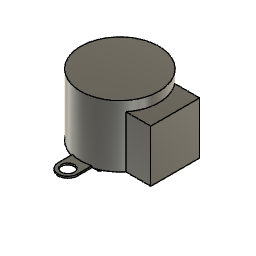
Moteur_Boule v1 (Autodesk Fusion 360 design; units mm, degrees)
Autodesk Fusion 360 part; units mm, degrees
sketch "Esquisse1" plane through (0, 0, 0) normal (0, 0, 1) x (1, 0, 0)
  circle A0 centre (0, 0) radius 12
  line L0 (9, 0) -> (17, 0)
  line L1 (17, -7.5) -> (9, -7.5)
  line L2 (9, -7.5) -> (9, 7.5)
  line L3 (9, 7.5) -> (17, 7.5)
  line L4 (17, 7.5) -> (17, -7.5)
  dimension "d1" = 24
  dimension "d3" = 8
  dimension "d4" = 17
  dimension "d5" = 15
  dimension "d8" = 7.5
  dimension "d9" = 8
  constraint coincident A0.centre origin
  constraint horizontal L0
  constraint horizontal L1
  constraint vertical L2
  constraint horizontal L3
  constraint vertical L4
  constraint collinear A0.centre L0.start L0.end
  constraint collinear L0.end L1.start L3.end
  measures "d1" diameter of A0
  measures "d3" distance of L0.start L0.end
  measures "d4" distance of A0.centre L0.end
  measures "d5" distance of L1 L3
  measures "d8" distance of L0 L1
  measures "d9" distance of L2.end L3.end
extrude "Extrusion1" add sketch "Esquisse1" along normal blind 16
sketch "Esquisse2" plane through (0, 0, 16) normal (0, 0, 1) x (-1, 0, 0)
  arc A0 (-9.3675, -7.5) -> (-9.3675, 7.5) centre (0, 0) ccw
  line L0 (-9.3675, 7.5) -> (-17, 7.5)
  line L1 (-17, 7.5) -> (-17, -7.5)
  line L2 (-17, -7.5) -> (-9.3675, -7.5)
  circle A1 centre (0, 0) radius 12
  constraint concentric A0 A1
extrude "Extrusion2" add sketch "Esquisse2" along normal blind 3 contours A0 A1
sketch "Esquisse5" plane through (0, 0, 0) normal (0, 0, -1) x (1, 0, 0)
  arc A0 (9.3675, 7.5) -> (9.3675, -7.5) centre (0, 0) ccw
  line L0 (9.3675, -7.5) -> (17, -7.5)
  line L1 (17, -7.5) -> (17, 7.5)
  line L2 (17, 7.5) -> (9.3675, 7.5)
  circle A1 centre (0, 16) radius 2
  line L3 (0, 0) -> (12, 0)
  circle A2 centre (0, 0) radius 12
  line L4 (3, 16) -> (3, 11.619)
  line L5 (0, 0) -> (0, 19)
  arc A3 (-3, -16) -> (0, -19) centre (0, -16) ccw
  line L6 (3, -16) -> (3, -11.619)
  circle A4 centre (0, -16) radius 2
  line L7 (-3, 16) -> (-3, 11.619)
  arc A5 (0, -19) -> (3, -16) centre (0, -16) ccw
  arc A6 (0, 19) -> (-3, 16) centre (0, 16) ccw
  line L8 (-3, 16) -> (3, 16)
  arc A7 (3, 16) -> (0, 19) centre (0, 16) ccw
  line L9 (-3, -16) -> (-3, -11.619)
  point P0 (0, 12)
  dimension "d27" = 19
  dimension "d28" = 4
  dimension "d29" = 24
  dimension "d30" = 3
  constraint coincident A0.centre L3.start
  constraint vertical L5
  constraint coincident A1.centre L5
  constraint coincident P0 L5
  constraint perpendicular L3 L5
  constraint coincident A1.centre A6.centre
  constraint perpendicular L5 L8
  constraint coincident L4.end A2
  constraint tangent L4 A7
  constraint coincident L7.end A2
  constraint tangent L7 A6
  constraint perpendicular L7 L8
  constraint symmetric A3.end L5.end L3
  constraint symmetric A1 L3 A4
  constraint symmetric L6.start L4.start L3
  constraint symmetric L3 A5 A7
  constraint symmetric A3.start L7.start L3
  constraint symmetric L3 A3 A6
  constraint symmetric L4.end L6.end L3
  constraint symmetric L7.end L9.end L3
  measures "d27" distance of A0.centre L5.end
  measures "d28" diameter of A1
  measures "d29" diameter of A2
  measures "d30" distance of L8 A7
extrude "Extrusion4" add sketch "Esquisse5" against normal blind 0.5 contours A0 A1 A2 L4 L5 L8 | A0 A1 A2 L5 L7 L8 | A1 L5 L8 A7 | A1 L5 A6 L8 | A0 A2 A3 L6 A5 L9
sketch "Esquisse6" plane through (0, 0, 0) normal (0, 0, -1) x (1, 0, 0)
  circle A0 centre (0, -16) radius 2
  circle A1 centre (0, 16) radius 2
  arc A2 (3, -11.619) -> (9.3675, -7.5) centre (0, 0) ccw
  line L0 (9.3675, -7.5) -> (17, -7.5)
  line L1 (17, -7.5) -> (17, 7.5)
  line L2 (17, 7.5) -> (9.3675, 7.5)
  arc A3 (9.3675, 7.5) -> (3, 11.619) centre (0, 0) ccw
  line L3 (3, 11.619) -> (3, 16)
  arc A4 (3, 16) -> (-3, 16) centre (0, 16) ccw
  line L4 (-3, 16) -> (-3, 11.619)
  arc A5 (-3, 11.619) -> (-3, -11.619) centre (0, 0) ccw
  line L5 (-3, -11.619) -> (-3, -16)
  arc A6 (-3, -16) -> (3, -16) centre (0, -16) ccw
  line L6 (3, -16) -> (3, -11.619)
  circle A7 centre (-7, 0) radius 4
  line L7 (-7, 0) -> (-12, 0)
  dimension "d33" = 8
  dimension "d34" = 5
  constraint coincident A7.centre L7.start
  constraint midpoint A5 L7.end
  constraint horizontal L7
  measures "d33" diameter of A7
  measures "d34" distance of A7.centre L7.end
extrude "Extrusion5" add sketch "Esquisse6" along normal blind 1 contours A7
sketch "Esquisse7" plane through (0, 0, -1) normal (0, 0, -1) x (1, 0, 0)
  circle A0 centre (-7, 0) radius 4
  circle A1 centre (-7, 0) radius 2.5
  dimension "d37" = 5
  constraint concentric A0 A1
  measures "d37" diameter of A1
extrude "Extrusion6" add sketch "Esquisse7" along normal blind 9 contours A1
sketch "Esquisse8" plane through (0, 0, -10) normal (0, 0, -1) x (1, 0, 0)
  circle A0 centre (-7, 0) radius 2.5
  line L0 (-7, 0) -> (-9.5, 0)
  line L1 (-7, 0) -> (-4.5, 0)
  line L2 (-9, 0) -> (-5, 0)
  line L3 (-5, 0) -> (-5, 1.5)
  line L4 (-5, 1.5) -> (-9, 1.5)
  line L5 (-9, 1.5) -> (-9, 0)
  line L6 (-5, -1.5) -> (-9, -1.5)
  line L7 (-9, -1.5) -> (-9, 0)
  line L8 (-5, 0) -> (-5, -1.5)
  dimension "d43" = 4
  dimension "d44" = 1.5
  dimension "d45" = 2
  constraint coincident A0.centre L0.start
  constraint coincident A0 L0.end
  constraint horizontal L0
  constraint coincident A0 L1.end
  constraint parallel L0 L1
  constraint horizontal L2
  constraint vertical L3
  constraint horizontal L4
  constraint vertical L5
  constraint coincident L0 L2.start
  constraint symmetric L5.end L2 L7.end
  constraint symmetric L3.start L2 L8.start
  constraint symmetric L3.end L2 L6.start
  constraint symmetric L4.end L2 L6.end
  measures "d43" distance of L3.end L4.end
  measures "d44" distance of L1 L4
  measures "d45" distance of A0.centre L5
extrude "Extrusion7" cut sketch "Esquisse8" against normal blind 6 contours A0 L4 | A0 L6
